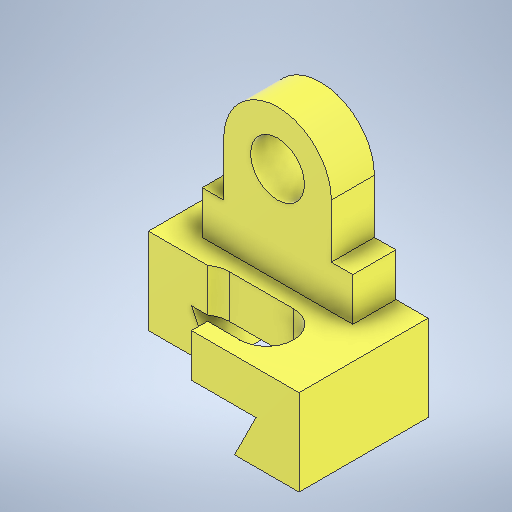
# Autodesk Inventor part: Деталь1-1
Saved by Autodesk Inventor 2025 (Build 290162000, 162)
## iProperties
Created: 2024-11-02
Part Number: Деталь1-1
Material: Типовые
Document SubType Name: Modeling
Designer: shoptick
Density: 1 g/cm^3
Appearance: По умолчанию
Author: shoptick
Autodesk Inventor part; units mm, degrees
ref_plane "XZ Plane" through (0, 0, 0) normal (0, 1, 0) x (-1, 0, 0)
sketch "Эскиз1" plane through (0, 0, 0) normal (0, 1, 0) x (-1, 0, 0)
  line L0 (0, 0) -> (-100, 0)
  line L1 (-100, 0) -> (-100, -60)
  line L2 (-100, -60) -> (0, -60)
  line L3 (0, -60) -> (0, 0)
  dimension "d0" = 100
  dimension "d1" = 60
  constraints: 8 end point, 2 parallel, 1 horizontal, 1 perpendicular
  measures "d0" distance of L2.end L1.end
  measures "d1" distance of L1.end L0.end
extrude "Выдавливание1" add sketch "Эскиз1" along normal blind 40
sketch "Эскиз2" plane through (0, 0, 0) normal (0, 0, 1) x (1, 0, 0)
  line L0 (100, 0) -> (0, 0) projected
  line L1 (0, 0) -> (0, 40) projected
  line L2 (0, 40) -> (100, 40) projected
  line L3 (100, 40) -> (100, 0) projected
  line L4 (50, 0) -> (30, 0)
  line L5 (50, 0) -> (50, 20)
  line L6 (50, 20) -> (20, 20)
  line L7 (20, 20) -> (30, 0)
  line L8 (50, 0) -> (70, 0)
  line L9 (50, 20) -> (80, 20)
  line L10 (80, 20) -> (70, 0)
  dimension "d5" = 20
  dimension "d6" = 20
  dimension "d7" = 30
  constraints: 14 end point, 2 symmetric about line, 1 horizontal, 1 midpoint, 1 perpendicular
  measures "d5" distance of L4.start L4.end
  measures "d6" distance of L4.start L5.end
  measures "d7" distance of L5.end L6.end
extrude "Выдавливание2" cut sketch "Эскиз2" against normal blind 60 contours L0 L5 L9 L10 | L0 L7 L6 L5
sketch "Эскиз3" plane through (100, 40, -60) normal (0, 0, -1) x (-1, 0, 0)
  line L0 (20, -20) -> (30, -40) projected
  line L1 (30, -40) -> (0, -40) projected
  line L2 (0, -40) -> (0, 0) projected
  line L3 (0, 0) -> (100, 0) projected
  line L4 (100, 0) -> (100, -40) projected
  line L5 (100, -40) -> (70, -40) projected
  line L6 (70, -40) -> (80, -20) projected
  line L7 (80, -20) -> (20, -20) projected
  line L8 (50, 0) -> (15, 0)
  arc A0 (50, 57.5) -> (50, 32.5) centre (50, 45) ccw
  arc A1 (50, 70) -> (25, 45) centre (50, 45) ccw
  line L9 (15, 0) -> (15, 20)
  line L10 (15, 20) -> (25, 20)
  line L11 (25, 20) -> (25, 45)
  line L12 (50, 0) -> (85, 0)
  arc A2 (50, 32.5) -> (50, 57.5) centre (50, 45) ccw
  arc A3 (75, 45) -> (50, 70) centre (50, 45) ccw
  line L13 (85, 0) -> (85, 20)
  line L14 (85, 20) -> (75, 20)
  line L15 (75, 20) -> (75, 45)
  dimension "d10" = 35
  dimension "d12" = 25
  dimension "d13" = 50
  dimension "d14" = 20
  dimension "d15" = 10
  constraints: 16 end point, 8 point on circle, 4 centre point, 2 coincident, 1 midpoint, 1 perpendicular, 1 point on line, 1 tangent, 1 vertical
  measures "d10" distance of L8.start L8.end
  measures "d12" diameter of A0
  measures "d13" diameter of A1
  measures "d14" distance of L8.end L9.end
  measures "d15" distance of L9.end L10.end
extrude "Выдавливание3" add sketch "Эскиз3" against normal blind 20 contours L9 L10 L11 A1 A3 L15 L14 L13 L3
sketch "Эскиз4" plane through (0, 40, 0) normal (0, 1, 0) x (1, 0, 0)
  line L0 (85, 40) -> (15, 40) projected
  arc A0 (35, 32.5) -> (35, 7.5) centre (35, 20) ccw
  line L1 (35, 32.5) -> (50, 32.5)
  line L2 (35, 7.5) -> (50, 7.5)
  arc A1 (65, 7.5) -> (65, 32.5) centre (65, 20) ccw
  line L3 (65, 32.5) -> (50, 32.5)
  line L4 (65, 7.5) -> (50, 7.5)
  point P0 (0, 0)
  dimension "d20" = 25
  constraints: 8 end point, 4 point on circle, 2 centre point, 2 horizontal
  measures "d20" diameter of A0
extrude "Выдавливание4" cut sketch "Эскиз4" against normal blind 20
ref_plane "РабПлоскость1" through (50, 0, 0) normal (1, 0, 0) x (0, 1, 0)
ref_plane "РабПлоскость2" through (0, 0, -30) normal (0, 0, 1) x (1, 0, 0)
split body "Разделение1" result two bodies by plane through (0, 0, -30) normal (0, 0, 1) first body at (60, 33.3333, -0.5)
split "Разделение2" plane through (50, 0, 0) removes the side toward (-1, 0, 0) bodies 2
combine bodies "Комбинировать1" operation type add bodies to combine 3 2
